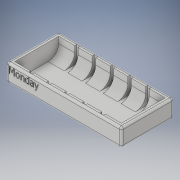
# Autodesk Inventor part: Monday
Saved by Autodesk Inventor 2019.4 (Build 234330000, 330)
## iProperties
Created: 2020-10-20
Part Number: Monday
Material: Generic
Document SubType Name: Modeling
Designer: daanswinters
Density: 1 g/cm^3
Appearance: Default
Author: daanswinters
Autodesk Inventor part; units mm, degrees
ref_plane "YZ Plane" through (0, 0, 0) normal (1, 0, 0) x (0, 1, 0)
ref_plane "XZ Plane" through (0, 0, 0) normal (0, 1, 0) x (-1, 0, 0)
ref_plane "XY Plane" through (0, 0, 0) normal (0, 0, 1) x (1, 0, 0)
sketch "Sketch1" plane through (0, 0, 0) normal (0, 0, 1) x (1, 0, 0)
  line L0 (55, -8.5) -> (-55, -8.5)
  line L1 (-55, -8.5) -> (-55, 8.5)
  line L2 (-55, 8.5) -> (55, 8.5)
  line L3 (55, 8.5) -> (55, -8.5)
  line L4 (55, -8.5) -> (-55, 8.5) construction
  line L5 (-55, -8.5) -> (55, 8.5) construction
  point P0 (0, 0)
  dimension "d0" = 110
  dimension "d1" = 17
  constraints: 12 end point, 2 midpoint, 2 parallel, 1 horizontal, 1 perpendicular
  measures "d0" distance of L1.end L2.end
  measures "d1" distance of L0.end L1.end
extrude "Extrusion1" add sketch "Sketch1" along normal blind 50
sketch "Sketch2" plane through (-55, 8.5, 0) normal (0, 1, 0) x (1, 0, 0)
  line L0 (0, 0) -> (0, -50) projected
  line L1 (110, -50) -> (0, -50)
  line L2 (0, -50) -> (0, 0)
  line L3 (0, 0) -> (110, 0)
  line L4 (110, 0) -> (110, -50)
  line L5 (110, -50) -> (0, 0) construction
  line L6 (0, -50) -> (110, 0) construction
  line L7 (106, -46) -> (106, -4)
  line L8 (4, -4) -> (4, -46)
  line L9 (56.15, -2) -> (53.85, -2)
  line L10 (53.85, -48) -> (56.15, -48)
  line L11 (56.15, -2) -> (53.85, -48) construction
  line L12 (53.85, -2) -> (56.15, -48) construction
  line L13 (73.15, -2) -> (70.85, -2)
  line L14 (70.85, -48) -> (73.15, -48)
  line L15 (73.15, -2) -> (70.85, -48) construction
  line L16 (70.85, -2) -> (73.15, -48) construction
  line L17 (0, -25) -> (110, -25) construction
  line L18 (87.85, -2) -> (90.15, -2)
  line L19 (90.15, -48) -> (87.85, -48)
  line L20 (87.85, -2) -> (90.15, -48) construction
  line L21 (90.15, -2) -> (87.85, -48) construction
  line L22 (36.85, -2) -> (39.15, -2)
  line L23 (39.15, -48) -> (36.85, -48)
  line L24 (36.85, -2) -> (39.15, -48) construction
  line L25 (39.15, -2) -> (36.85, -48) construction
  line L26 (19.85, -2) -> (22.15, -2)
  line L27 (22.15, -48) -> (19.85, -48)
  line L28 (19.85, -2) -> (22.15, -48) construction
  line L29 (22.15, -2) -> (19.85, -48) construction
  line L30 (90.15, -2) -> (90.15, -4)
  line L31 (90.15, -46) -> (90.15, -48)
  line L32 (87.85, -48) -> (87.85, -46)
  line L33 (87.85, -4) -> (87.85, -2)
  line L34 (73.15, -48) -> (73.15, -46)
  line L35 (73.15, -4) -> (73.15, -2)
  line L36 (70.85, -2) -> (70.85, -4)
  line L37 (70.85, -46) -> (70.85, -48)
  line L38 (56.15, -4) -> (56.15, -2)
  line L39 (53.85, -2) -> (53.85, -4)
  line L40 (53.85, -46) -> (53.85, -48)
  line L41 (56.15, -48) -> (56.15, -46)
  line L42 (39.15, -2) -> (39.15, -4)
  line L43 (39.15, -46) -> (39.15, -48)
  line L44 (36.85, -48) -> (36.85, -46)
  line L45 (36.85, -4) -> (36.85, -2)
  line L46 (22.15, -2) -> (22.15, -4)
  line L47 (19.85, -48) -> (19.85, -46)
  line L48 (19.85, -4) -> (19.85, -2)
  line L49 (22.15, -46) -> (22.15, -48)
  line L50 (4, -46) -> (19.95, -46)
  line L51 (22.05, -46) -> (36.95, -46)
  line L52 (39.05, -46) -> (53.95, -46)
  line L53 (56.05, -46) -> (70.95, -46)
  line L54 (73.05, -46) -> (87.95, -46)
  line L55 (90.05, -46) -> (106, -46)
  line L56 (106, -4) -> (90.05, -4)
  line L57 (87.95, -4) -> (73.05, -4)
  line L58 (70.95, -4) -> (56.05, -4)
  line L59 (53.95, -4) -> (39.05, -4)
  line L60 (36.95, -4) -> (22.05, -4)
  line L61 (19.95, -4) -> (4, -4)
  point P0 (55, 0)
  point P1 (55, -25)
  point P2 (72, -25)
  point P3 (89, -25)
  point P4 (38, -25)
  point P5 (21, -25)
  dimension "d4" = 65.556
  dimension "d5" = 110
  dimension "d7" = 2.3
  dimension "d8" = 46
  dimension "d9" = 2.3
  dimension "d10" = 46
  dimension "d11" = 0
  dimension "d12" = 2.3
  dimension "d13" = 46
  dimension "d14" = 2.3
  dimension "d15" = 46
  dimension "d16" = 2.3
  dimension "d17" = 46
  dimension "d18" = 17
  dimension "d19" = 17
  dimension "d20" = 17
  dimension "d21" = 17
  dimension "d22" = 2.862
  dimension "d23" = 2.862
  dimension "d24" = 106
  dimension "d25" = 4
  dimension "d26" = 42
  dimension "d27" = 2
  dimension "d28" = 0
  dimension "d29" = 42
  dimension "d30" = 0
  dimension "d31" = 42
  dimension "d32" = 0
  dimension "d33" = 42
  dimension "d34" = 0
  dimension "d35" = 42
  dimension "d36" = 0
  dimension "d37" = 42
  constraints: 122 end point, 73 parallel, 43 point on line, 17 perpendicular, 14 midpoint, 6 horizontal
  measures "d4" angle of L5 L0
  measures "d5" distance between parallel lines of L4 L0
  measures "d7" distance of L10.end L10.start
  measures "d8" distance of L10.start L9.end
  measures "d9" distance of L14.end L14.start
  measures "d10" distance of L14.start L13.end
  measures "d11" distance from line of L17 point (72, -25)
  measures "d12" distance of L19.start L19.end
  measures "d13" distance of L18.end L19.start
  measures "d14" distance of L23.start L23.end
  measures "d15" distance of L22.end L23.start
  measures "d16" distance of L27.start L27.end
  measures "d17" distance of L26.end L27.start
  measures "d18" distance of point (72, -25) point (55, -25)
  measures "d19" distance of point (89, -25) point (72, -25)
  measures "d20" distance of point (38, -25) point (55, -25)
  measures "d21" distance of point (21, -25) point (38, -25)
  measures "d22" angle of L0 L20
  measures "d23" angle of L0 L21
  measures "d24" distance between parallel lines of L7 L0
  measures "d25" distance between parallel lines of L8 L0
  measures "d26" distance between parallel lines of L56 L55
  measures "d27" distance between parallel lines of L56 L18
  measures "d28" distance between parallel lines of L56 L57
  measures "d29" distance between parallel lines of L56 L54
  measures "d30" distance between parallel lines of L56 L58
  measures "d31" distance between parallel lines of L56 L53
  measures "d32" distance between parallel lines of L56 L59
  measures "d33" distance between parallel lines of L56 L52
  measures "d34" distance between parallel lines of L56 L60
  measures "d35" distance between parallel lines of L56 L51
  measures "d36" distance between parallel lines of L56 L61
  measures "d37" distance between parallel lines of L56 L50
extrude "Extrusion2" cut sketch "Sketch2" against normal blind 16 contours L55 L31 L19 L32 L54 L34 L14 L37 L53 L41 L10 L40 L52 L43 L23 L44 L51 L49 L27 L47 L50 L8 L61 L48 L26 L46 L60 L45 L22 L42 L59 L39 L9 L38 L58 L36 L13 L35 L57 L33 L18 L30 L56 L7
fillet "Fillet1" radius 2 12 edges at (-55, 0, 50) (-55, 0, 0) (55, 0, 50) (55, 0, 0) (0, 8.5, 50) (-55, 8.5, 25) (0, 8.5, 0) (55, 8.5, 25) (55, -8.5, 25) (0, -8.5, 50) (-55, -8.5, 25) (0, -8.5, 0)
fillet "Fillet2" radius 10 6 edges at (-43.075, -7.5, 4) (-25.5, -7.5, 4) (-8.5, -7.5, 4) (8.5, -7.5, 4) (25.5, -7.5, 4) (43.075, -7.5, 4)
sketch "Sketch3" plane through (35.15, 8.5, 4) normal (0, 1, 0) x (1, 0, 0)
  line L0 (-70.3, -44) -> (-70.3, -42) projected
  line L1 (-51, 2) -> (-53.3, 2)
  line L2 (-34, 2) -> (-34, 0) projected
  line L3 (-36.3, -44) -> (-36.3, -42) projected
  line L4 (-19.3, -44) -> (-19.3, -42) projected
  line L5 (-2.3, -44) -> (-2.3, -42) projected
  line L6 (0, 2) -> (0, 0) projected
  line L7 (-19.8, 2) -> (-16.5, 2)
  line L8 (-16.5, 2) -> (-16.5, -44)
  line L9 (-16.5, -44) -> (-19.8, -44)
  line L10 (-19.8, -44) -> (-19.8, 2)
  line L11 (-19.8, 2) -> (-16.5, -44) construction
  line L12 (-16.5, 2) -> (-19.8, -44) construction
  line L13 (-2.8, -44) -> (0.5, -44)
  line L14 (0.5, -44) -> (0.5, 2)
  line L15 (0.5, 2) -> (-2.8, 2)
  line L16 (-2.8, 2) -> (-2.8, -44)
  line L17 (-2.8, -44) -> (0.5, 2) construction
  line L18 (0.5, -44) -> (-2.8, 2) construction
  line L19 (-36.8, -44) -> (-33.5, -44)
  line L20 (-33.5, -44) -> (-33.5, 2)
  line L21 (-33.5, 2) -> (-36.8, 2)
  line L22 (-36.8, 2) -> (-36.8, -44)
  line L23 (-36.8, -44) -> (-33.5, 2) construction
  line L24 (-33.5, -44) -> (-36.8, 2) construction
  line L25 (-51, 2) -> (-36.3, 2) projected
  line L26 (-53.8, -44) -> (-50.5, -44)
  line L27 (-50.5, -44) -> (-50.5, 2)
  line L28 (-50.5, 2) -> (-53.8, 2)
  line L29 (-53.8, 2) -> (-53.8, -44)
  line L30 (-53.8, -44) -> (-50.5, 2) construction
  line L31 (-50.5, -44) -> (-53.8, 2) construction
  line L32 (-53.3, -44) -> (-68, -44) projected
  line L33 (-70.8, 2) -> (-67.5, 2)
  line L34 (-67.5, 2) -> (-67.5, -44)
  line L35 (-67.5, -44) -> (-70.8, -44)
  line L36 (-70.8, -44) -> (-70.8, 2)
  line L37 (-70.8, 2) -> (-67.5, -44) construction
  line L38 (-67.5, 2) -> (-70.8, -44) construction
  point P0 (-35.15, 4)
  point P1 (-68, 2)
  point P2 (-17, 2)
  point P3 (-18.15, -21)
  point P4 (-1.15, -21)
  point P5 (-35.15, -21)
  point P6 (-52.15, -21)
  point P7 (-69.15, -21)
  dimension "d42" = 3.3
  dimension "d43" = 46
  dimension "d44" = 3.3
  dimension "d45" = 3.3
  dimension "d46" = 3.3
  dimension "d47" = 3.3
  dimension "d48" = 90
  dimension "d49" = 0.5
  dimension "d50" = 16.5
  dimension "d51" = 33.5
  dimension "d52" = 50.5
  dimension "d53" = 67.5
  dimension "d54" = 46
  dimension "d55" = 0
  dimension "d56" = 53.3
  constraints: 62 end point, 14 parallel, 10 midpoint, 5 horizontal, 5 perpendicular, 3 point on line
  measures "d42" distance of L8.end L9.end
  measures "d43" distance of L7.end L8.end
  measures "d44" distance of L15.end L14.end
  measures "d45" distance of L21.end L20.end
  measures "d46" distance of L28.end L27.end
  measures "d47" distance of L34.end L35.end
  measures "d48" angle of L6 L1
  measures "d49" distance between parallel lines of L6 L14
  measures "d50" distance between parallel lines of L6 L8
  measures "d51" distance between parallel lines of L6 L20
  measures "d52" distance between parallel lines of L6 L27
  measures "d53" distance between parallel lines of L6 L34
  measures "d54" distance between parallel lines of L25 L9
  measures "d55" distance between parallel lines of L15 L25
  measures "d56" distance from line of L1.end L6
extrude "Extrusion3" cut sketch "Sketch3" against normal blind 16
sketch "Sketch4" plane through (0, 0, 50) normal (0, 0, 1) x (1, 0, 0)
  line L0 (-52.9749, 6.5012) -> (53.0345, 6.5012) construction
  line L1 (53.0345, 6.5012) -> (53.0345, -6.5247) construction
  line L2 (53.0345, -6.5247) -> (-52.9749, -6.5247) construction
  line L3 (-52.9749, -6.5247) -> (-52.9749, 6.5012) construction
  line L4 (-47.127, 0.1294) -> (-47.9377, 0.1294)
  line L5 (-47.9377, 0.1294) -> (-47.9377, 5.3841)
  line L6 (-47.9377, 5.3841) -> (-49.5295, 1.8101)
  line L7 (-49.5295, 1.8101) -> (-50.0238, 1.8101)
  line L8 (-50.0238, 1.8101) -> (-51.6007, 5.3841)
  line L9 (-51.6007, 5.3841) -> (-51.6007, 0.1294)
  line L10 (-51.6007, 0.1294) -> (-52.357, 0.1294)
  line L11 (-52.357, 0.1294) -> (-52.357, 6.2294)
  line L12 (-52.357, 6.2294) -> (-51.2497, 6.2294)
  line L13 (-51.2497, 6.2294) -> (-49.7272, 2.8333)
  line L14 (-49.7272, 2.8333) -> (-48.2541, 6.2294)
  line L15 (-48.2541, 6.2294) -> (-47.127, 6.2294)
  line L16 (-47.127, 6.2294) -> (-47.127, 0.1294)
  spline S0 degree 2 poles (-42.1887, 2.4181) (-42.1887, 1.2614) (-43.3009, 0.0008) (-44.2303, 0.0008) knots 0 0 0 1 2 2 2
  spline S1 degree 2 poles (-44.2303, 0.0008) (-45.1843, 0.0008) (-46.2768, 1.3009) (-46.2768, 2.4181) knots 0 0 0 1 2 2 2
  spline S2 degree 2 poles (-46.2768, 2.4181) (-46.2768, 3.5649) (-45.1497, 4.8354) (-44.2303, 4.8354) knots 0 0 0 1 2 2 2
  spline S3 degree 2 poles (-44.2303, 4.8354) (-43.3009, 4.8354) (-42.1887, 3.5699) (-42.1887, 2.4181) knots 0 0 0 1 2 2 2
  spline S4 degree 2 poles (-42.9846, 2.4181) (-42.9846, 3.3079) (-43.6321, 4.173) (-44.2303, 4.173) knots 0 0 0 1 2 2 2
  spline S5 degree 2 poles (-44.2303, 4.173) (-44.8284, 4.173) (-45.4809, 3.3079) (-45.4809, 2.4181) knots 0 0 0 1 2 2 2
  spline S6 degree 2 poles (-45.4809, 2.4181) (-45.4809, 1.553) (-44.8284, 0.6632) (-44.2303, 0.6632) knots 0 0 0 1 2 2 2
  spline S7 degree 2 poles (-44.2303, 0.6632) (-43.6371, 0.6632) (-42.9846, 1.5382) (-42.9846, 2.4181) knots 0 0 0 1 2 2 2
  line L17 (-37.804, 0.1294) -> (-38.5752, 0.1294)
  line L18 (-38.5752, 0.1294) -> (-38.5752, 2.7394)
  spline S8 degree 2 poles (-38.5752, 2.7394) (-38.5752, 3.0558) (-38.6345, 3.5995) (-38.7235, 3.7627) knots 0 0 0 1 2 2 2
  spline S9 degree 2 poles (-38.7235, 3.7627) (-38.8174, 3.9357) (-39.1535, 4.1038) (-39.4402, 4.1038) knots 0 0 0 1 2 2 2
  spline S10 degree 2 poles (-39.4402, 4.1038) (-39.727, 4.1038) (-40.335, 3.7973) (-40.6266, 3.5501) knots 0 0 0 1 2 2 2
  line L19 (-40.6266, 3.5501) -> (-40.6266, 0.1294)
  line L20 (-40.6266, 0.1294) -> (-41.3978, 0.1294)
  line L21 (-41.3978, 0.1294) -> (-41.3978, 4.7068)
  line L22 (-41.3978, 4.7068) -> (-40.6266, 4.7068)
  line L23 (-40.6266, 4.7068) -> (-40.6266, 4.1977)
  spline S11 degree 2 poles (-40.6266, 4.1977) (-40.2806, 4.5091) (-39.6133, 4.8354) (-39.2376, 4.8354) knots 0 0 0 1 2 2 2
  spline S12 degree 2 poles (-39.2376, 4.8354) (-38.5653, 4.8354) (-37.804, 3.9456) (-37.804, 3.1003) knots 0 0 0 1 2 2 2
  line L24 (-37.804, 3.1003) -> (-37.804, 0.1294)
  line L25 (-33.2018, 0.1294) -> (-33.973, 0.1294)
  line L26 (-33.973, 0.1294) -> (-33.973, 0.594)
  spline S13 degree 2 poles (-33.973, 0.594) (-34.1509, 0.4457) (-34.4129, 0.248) (-34.5909, 0.164) knots 0 0 0 1 2 2 2
  spline S14 degree 2 poles (-34.5909, 0.164) (-34.754, 0.0849) (-35.105, 0.0008) (-35.3373, 0.0008) knots 0 0 0 1 2 2 2
  spline S15 degree 2 poles (-35.3373, 0.0008) (-35.713, 0.0008) (-36.3458, 0.3123) (-36.5682, 0.6138) knots 0 0 0 1 2 2 2
  spline S16 degree 2 poles (-36.5682, 0.6138) (-36.7906, 0.9153) (-37.0378, 1.8051) (-37.0378, 2.3835) knots 0 0 0 1 2 2 2
  spline S17 degree 2 poles (-37.0378, 2.3835) (-37.0378, 2.9866) (-36.7264, 3.8665) (-36.4545, 4.1977) knots 0 0 0 1 2 2 2
  spline S18 degree 2 poles (-36.4545, 4.1977) (-36.2024, 4.4943) (-35.4955, 4.8354) (-35.105, 4.8354) knots 0 0 0 1 2 2 2
  spline S19 degree 2 poles (-35.105, 4.8354) (-34.7639, 4.8354) (-34.2547, 4.6821) (-33.973, 4.5239) knots 0 0 0 1 2 2 2
  line L27 (-33.973, 4.5239) -> (-33.973, 6.5012)
  line L28 (-33.973, 6.5012) -> (-33.2018, 6.5012)
  line L29 (-33.2018, 6.5012) -> (-33.2018, 0.1294)
  line L30 (-33.973, 1.2416) -> (-33.973, 3.8863)
  spline S20 degree 2 poles (-33.973, 3.8863) (-34.2597, 4.0247) (-34.7145, 4.1285) (-34.9765, 4.1285) knots 0 0 0 1 2 2 2
  spline S21 degree 2 poles (-34.9765, 4.1285) (-35.5697, 4.1285) (-36.2419, 3.2387) (-36.2419, 2.3983) knots 0 0 0 1 2 2 2
  spline S22 degree 2 poles (-36.2419, 2.3983) (-36.2419, 1.5876) (-35.7278, 0.7324) (-35.1594, 0.7324) knots 0 0 0 1 2 2 2
  spline S23 degree 2 poles (-35.1594, 0.7324) (-34.8578, 0.7324) (-34.2449, 1.0093) (-33.973, 1.2416) knots 0 0 0 1 2 2 2
  spline S24 degree 2 poles (-29.5339, 0.6138) (-29.6278, 0.5446) (-29.9442, 0.2974) (-30.0925, 0.2233) knots 0 0 0 1 2 2 2
  spline S25 degree 2 poles (-30.0925, 0.2233) (-30.2952, 0.1145) (-30.6758, 0.0008) (-31.0218, 0.0008) knots 0 0 0 1 2 2 2
  spline S26 degree 2 poles (-31.0218, 0.0008) (-31.3036, 0.0008) (-31.8128, 0.2134) (-32.0056, 0.4062) knots 0 0 0 1 2 2 2
  spline S27 degree 2 poles (-32.0056, 0.4062) (-32.1885, 0.594) (-32.4109, 1.1477) (-32.4109, 1.4542) knots 0 0 0 1 2 2 2
  spline S28 degree 2 poles (-32.4109, 1.4542) (-32.4109, 1.9287) (-32.0105, 2.601) (-31.5755, 2.7938) knots 0 0 0 1 2 2 2
  spline S29 degree 2 poles (-31.5755, 2.7938) (-31.1899, 2.9718) (-30.1419, 3.1052) (-29.5339, 3.1398) knots 0 0 0 1 2 2 2
  line L31 (-29.5339, 3.1398) -> (-29.5339, 3.2881)
  spline S30 degree 2 poles (-29.5339, 3.2881) (-29.5339, 3.5551) (-29.697, 3.8863) (-29.8453, 3.9802) knots 0 0 0 1 2 2 2
  spline S31 degree 2 poles (-29.8453, 3.9802) (-29.9936, 4.0741) (-30.4188, 4.1334) (-30.6462, 4.1334) knots 0 0 0 1 2 2 2
  spline S32 degree 2 poles (-30.6462, 4.1334) (-30.9131, 4.1334) (-31.6348, 3.9752) (-31.9957, 3.822) knots 0 0 0 1 2 2 2
  line L32 (-31.9957, 3.822) -> (-32.0402, 3.822)
  line L33 (-32.0402, 3.822) -> (-32.0402, 4.608)
  spline S33 degree 2 poles (-32.0402, 4.608) (-31.8276, 4.6673) (-31.0317, 4.8156) (-30.6412, 4.8156) knots 0 0 0 1 2 2 2
  spline S34 degree 2 poles (-30.6412, 4.8156) (-30.1667, 4.8156) (-29.5191, 4.6673) (-29.262, 4.4745) knots 0 0 0 1 2 2 2
  spline S35 degree 2 poles (-29.262, 4.4745) (-29.0099, 4.2867) (-28.7628, 3.6885) (-28.7628, 3.2585) knots 0 0 0 1 2 2 2
  line L34 (-28.7628, 3.2585) -> (-28.7628, 0.1294)
  line L35 (-28.7628, 0.1294) -> (-29.5339, 0.1294)
  line L36 (-29.5339, 0.1294) -> (-29.5339, 0.6138)
  line L37 (-29.5339, 1.2564) -> (-29.5339, 2.5269)
  spline S36 degree 2 poles (-29.5339, 2.5269) (-29.8107, 2.5021) (-30.6462, 2.4181) (-30.9082, 2.339) knots 0 0 0 1 2 2 2
  spline S37 degree 2 poles (-30.9082, 2.339) (-31.2146, 2.2451) (-31.615, 1.8546) (-31.615, 1.5085) knots 0 0 0 1 2 2 2
  spline S38 degree 2 poles (-31.615, 1.5085) (-31.615, 1.1131) (-31.1701, 0.7127) (-30.745, 0.7127) knots 0 0 0 1 2 2 2
  spline S39 degree 2 poles (-30.745, 0.7127) (-30.3842, 0.7127) (-29.791, 1.0241) (-29.5339, 1.2564) knots 0 0 0 1 2 2 2
  line L38 (-24.0864, 4.7068) -> (-26.5482, -1.5563)
  line L39 (-26.5482, -1.5563) -> (-27.3737, -1.5563)
  line L40 (-27.3737, -1.5563) -> (-26.5531, 0.3518)
  line L41 (-26.5531, 0.3518) -> (-28.2141, 4.7068)
  line L42 (-28.2141, 4.7068) -> (-27.3836, 4.7068)
  line L43 (-27.3836, 4.7068) -> (-26.1329, 1.3158)
  line L44 (-26.1329, 1.3158) -> (-24.8872, 4.7068)
  line L45 (-24.8872, 4.7068) -> (-24.0864, 4.7068)
  point P0 (0, 0)
  constraints: 2 other
extrude "Extrusion4" cut sketch "Sketch4" against normal blind 0.5
fillet "Fillet3" radius 10 6 edges at (-43.325, -7.5, 46) (-25.5, -7.5, 46) (-8.5, -7.5, 46) (8.5, -7.5, 46) (25.5, -7.5, 46) (43.325, -7.5, 46)
body "Solid1"
